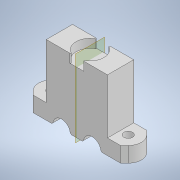
# Autodesk Inventor part: Magnet Mount
Saved by Autodesk Inventor 2022 (Build 260153000, 153)
## iProperties
Created: 2022-04-23
Part Number: Magnet Mount
Material: Generic
Document SubType Name: Modeling
Designer: Nick
Density: 1 g/cm^3
Appearance: Default
Author: Nick
Autodesk Inventor part; units mm, degrees
ref_plane "YZ Plane" through (0, 0, 0) normal (1, 0, 0) x (0, 1, 0)
ref_plane "XZ Plane" through (0, 0, 0) normal (0, 1, 0) x (-1, 0, 0)
ref_plane "XY Plane" through (0, 0, 0) normal (0, 0, 1) x (1, 0, 0)
sketch "Sketch1" plane through (0, 0, 0) normal (0, 0, 1) x (1, 0, 0)
  line L0 (0, 0) -> (28, 0)
  line L1 (28, 0) -> (28, 32)
  line L2 (28, 32) -> (0, 32)
  line L3 (0, 32) -> (0, 0)
  circle A0 centre (7, 0) radius 4
  circle A1 centre (21, 0) radius 4
  point P0 (3, 0)
  point P1 (11, 0)
  point P2 (17, 0)
  point P3 (25, 0)
  dimension "d0" = 28
  dimension "d1" = 32
  dimension "d2" = 8
  dimension "d3" = 8
  dimension "d4" = 14
  dimension "d5" = 7
  dimension "d6" = 7
  constraints: 8 end point, 2 centre point, 2 parallel, 2 point on line, 1 horizontal, 1 perpendicular
  measures "d0" distance of L2.end L1.end
  measures "d1" distance of L1.end L0.end
  measures "d2" diameter of A0
  measures "d3" diameter of A1
  measures "d4" distance of A0.centre A1.centre
  measures "d5" distance of L0.end A1.centre
  measures "d6" distance from line of L3 A0.centre
extrude "Extrusion1" add sketch "Sketch1" along normal blind 12 contours A1 L0 A0 L3 L2 L1
chamfer "Chamfer1" distance 0.5 angle 45 4 edges at (3, 0, 6) (11, 0, 6) (17, 0, 6) (25, 0, 6)
sketch "Sketch2" plane through (0, 32, 0) normal (0, 1, 0) x (1, 0, 0)
  circle A0 centre (14, -6) radius 6.35
  line L0 (28, 0) -> (0, 0) projected
  line L1 (28, 0) -> (28, -12) projected
  point P0 (14, 0)
  point P1 (28, -6)
  point P2 (16.0791, 0)
  point P3 (11.9209, 0)
  dimension "d12" = 12.7
  constraints: 2 midpoint, 1 centre point, 1 horizontal alignment, 1 vertical alignment
  measures "d12" diameter of A0
extrude "Extrusion2" cut sketch "Sketch2" against normal blind 4 contours A0 L0 picked at (13.6383, -8.0675)
fillet "Fillet1" radius 0.25 4 edges at (11.9209, 30, 0) (16.0791, 30, 0) (16.0791, 30, 12) (11.9209, 30, 12)
ref_plane "Work Plane3" through (14, 0, 0) normal (-1, 0, 0) x (0, 0, 1)
sketch "Sketch5" plane through (0, 0, 0) normal (0, -1, 0) x (1, 0, 0)
  circle A0 centre (-3.5, 6) radius 2
  circle A1 centre (-3.5, 6) radius 3.5
  circle A2 centre (-3.5, 6) radius 6
  line L0 (2.5, 12) -> (2.5, 0) projected
  line L1 (0, 12) -> (2.5, 12) projected
  line L2 (0, 0) -> (0, 12) projected
  line L3 (0, 0) -> (2.5, 0) projected
  line L4 (0, 0) -> (0, 12) projected
  line L5 (0, 0) -> (-5.9853, 0)
  line L6 (-5.9853, 0) -> (-7.7426, 1.7574)
  line L7 (0, 12) -> (-5.9853, 12)
  line L8 (-5.9853, 12) -> (-7.7426, 10.2426)
  line L9 (0, 0) -> (0, 12) projected
  dimension "d22" = 4
  dimension "d23" = 7
  dimension "d24" = 135
  dimension "d25" = 135
  constraints: 8 end point, 5 tangent, 3 centre point, 2 coincident, 2 horizontal, 2 point on circle
  measures "d22" diameter of A0
  measures "d23" diameter of A1
  measures "d24" angle of L7 L8
  measures "d25" angle of L5 L6
extrude "Extrusion3" add sketch "Sketch5" against normal blind 7 contours A0 | A1 | L2 A2 | L2 L5 A2 | A2 L7 L2 | L5 L6 A2 | A2 L8 L7 picked at (-7.4809, 9.2519)
sketch "Sketch6" plane through (2.5, 0, 0) normal (0, -1, 0) x (1, 0, 0)
  arc A0 (-10.2426, 10.2426) -> (-10.2426, 1.7574) centre (-6, 6) ccw projected
  point P0 (-2.5, 0)
hole "Hole1" at (-3.5, 0, 6) direction (0, 1, 0) diameter 4 end through all
mirror "Mirror2" about plane through (14, 0, 0) normal (-1, 0, 0) of "Extrusion3", "Hole1"
equation "\"d1\" = MotorHeight"
equation "\"d5\" = d6"
equation "\"MotorHeight\" = MotorHeightBase"
equation "\"MotorHeightBase\" = 32"
body "Solid1"
